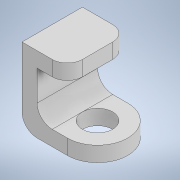
# Autodesk Inventor part: Exercise_3
Saved by Autodesk Inventor 2020 (Build 240168000, 168)
## iProperties
Created: 2022-11-07
Part Number: Exercise_3
Material: Generic
Document SubType Name: Modeling
Designer: Matthew Ng
Density: 1 g/cm^3
Appearance: Default
Author: Matthew Ng
Autodesk Inventor part; units mm, degrees
note: some values were not read from the file. Chosen so that the rebuilt part matches the saved one: direction of "Hole1".
ref_plane "YZ Plane" through (0, 0, 0) normal (1, 0, 0) x (0, 1, 0)
ref_plane "XZ Plane" through (0, 0, 0) normal (0, 1, 0) x (-1, 0, 0)
ref_plane "XY Plane" through (0, 0, 0) normal (0, 0, 1) x (1, 0, 0)
sketch "Sketch1" plane through (0, 0, 0) normal (0, 0, 1) x (1, 0, 0)
  line L0 (0, 60.4862) -> (0, -12.4973) projected
  line L1 (-12.4853, 0) -> (60.4142, 0) projected
  line L2 (0, 50.06) -> (30, 50.06)
  line L3 (30, 50.06) -> (30, 40.06)
  line L4 (30, 40.06) -> (10, 40.06)
  line L5 (0, 40.06) -> (0, 50.06)
  line L6 (10, 0) -> (50, 0)
  line L7 (50, 0) -> (50, 10)
  line L8 (50, 10) -> (20, 10)
  line L9 (0, 10) -> (0, 10)
  line L10 (10, 40.06) -> (10, 20)
  line L11 (0, 10) -> (0, 40.06)
  arc A0 (0, 10) -> (10, 0) centre (10, 10) ccw
  arc A1 (10, 20) -> (20, 10) centre (20, 20) ccw
  point P0 (0, 0)
  dimension "d0" = 30
  dimension "d2" = 50
  dimension "d3" = 10
  dimension "d5" = 10
  dimension "d6" = 10
  constraints: 20 end point, 5 parallel, 4 point on circle, 4 tangent, 3 point on line, 2 centre point, 2 horizontal, 2 perpendicular, 1 equal radius
  measures "d0" distance of L3.end L5.start
  measures "d2" distance of L9.start L7.end
  measures "d3" distance of L7.end L6.end
  measures "d5" radius of A0
  measures "d6" distance between parallel lines of L4 L2
extrude "Extrusion1" add sketch "Sketch1" along normal mid plane 40 contours L2 L3 L4 L10 A1 L8 L7 L1 A0 L0
fillet "Fillet1" radius 20 2 edges at (50, 5, 20) (50, 5, -20)
fillet "Fillet2" radius 10 2 edges at (30, 45.06, 20) (30, 45.06, -20)
sketch "Sketch2" plane through (10, 0, -20) normal (0, -1, 0) x (1, 0, 0)
  arc A0 (20, 0) -> (20, 40) centre (20, 20) ccw projected
  point P0 (-10, 20)
  constraints: 1 coincident
hole "Hole1" at (30, 0, 0) direction (0, 1, 0) diameter 20 depth 10
body "Solid1"
